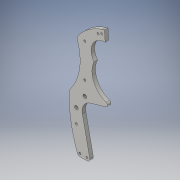
# Autodesk Inventor part: One piece claw 1.0
Saved by Autodesk Inventor 2016 (Build 200138000, 138)
## iProperties
Created: 2016-02-02
Part Number: One piece claw 1.0
Material: Generic
Document SubType Name: Modeling
Designer: Josiah Stark
Density: 1 g/cm^3
Appearance: Default
Author: Josiah Stark
Autodesk Inventor part; units mm, degrees
ref_plane "YZ Plane" through (0, 0, 0) normal (1, 0, 0) x (0, 1, 0)
ref_plane "XZ Plane" through (0, 0, 0) normal (0, 1, 0) x (-1, 0, 0)
ref_plane "XY Plane" through (0, 0, 0) normal (0, 0, 1) x (1, 0, 0)
sketch "Sketch1" plane through (0, 0, 0) normal (0, 0, 1) x (1, 0, 0)
  line L0 (-50.8, -25.4) -> (76.2, -25.4)
  line L1 (76.2, -25.4) -> (76.2, 228.6)
  line L2 (76.2, 228.6) -> (-51.6296, 228.6)
  circle A0 centre (5.08, -4.9022) radius 1.905
  circle A1 centre (-1.27, 63.6778) radius 3.175
  circle A2 centre (13.97, 89.0778) radius 3.175
  arc A3 (23.4649, 83.1687) -> (9.3315, 59.465) centre (29.21, 63.6778) ccw
  arc A4 (0.3002, -6.6225) -> (5.08, -9.9822) centre (5.08, -4.9022) ccw
  line L3 (5.08, -9.9822) -> (17.78, -9.9822)
  arc A5 (17.78, -9.9822) -> (22.7496, -3.849) centre (17.78, -4.9022) ccw
  line L4 (9.3315, 59.465) -> (22.7496, -3.849)
  arc A6 (-14.6784, 83.2471) -> (0.3002, -6.6225) centre (239.2924, 79.3933) ccw
  arc A7 (50.546, 191.9478) -> (30.3529, 151.1401) centre (50.546, 166.5478) ccw
  line L5 (50.546, 191.9478) -> (50.546, 210.9978)
  arc A8 (0.9197, 176.5759) -> (0.1225, 170.7438) centre (6.096, 172.8978) ccw
  arc A9 (50.546, 210.9978) -> (0.9197, 176.5759) centre (73.3878, 125.0824) ccw
  arc A10 (-13.9866, 85.1779) -> (0.1225, 170.7438) centre (-83.5064, 140.5873) ccw
  arc A11 (-13.9866, 85.1779) -> (-14.6784, 83.2471) centre (-11.5038, 83.199) ccw
  circle A12 centre (17.78, -4.9022) radius 1.905
  arc A13 (76.2, 171.1429) -> (75.486, 171.3598) centre (64.77, 134.7978) ccw
  arc A14 (30.3529, 151.1401) -> (52.1919, 98.8339) centre (64.77, 134.7978) ccw
  line L6 (-51.6296, 228.6) -> (-51.6296, 223.5757)
  line L7 (-50.8, -9.9822) -> (-50.8, -25.4)
  line L8 (45.5539, 209.5127) -> (50.546, 210.9978)
  arc A15 (55.9788, 92.7525) -> (55.982, 92.7794) centre (50.3052, 93.4393) ccw
  line L9 (48.0499, 210.2553) -> (50.546, 210.9978)
  line L10 (49.298, 210.6265) -> (50.546, 191.9478)
  line L11 (49.298, 210.6265) -> (49.1762, 210.5903)
  line L12 (49.1762, 210.5903) -> (50.546, 191.9478)
  arc A16 (51.9893, 91.5765) -> (52.1919, 98.8339) centre (50.9341, 95.2375) ccw
  line L13 (45.9382, 89.7529) -> (52.0334, 91.5895)
  line L14 (52.0334, 91.5895) -> (23.4649, 83.1687)
  circle A17 centre (13.97, 114.4778) radius 1.905
  circle A18 centre (13.97, 175.4378) radius 1.905
  circle A19 centre (44.6762, 202.1078) radius 1.905
  circle A20 centre (37.7491, 198.9328) radius 1.905
  circle A21 centre (-1.27, 38.2778) radius 1.905
  point P0 (0, 0)
  point P1 (50.546, 87.6896)
  dimension "d1" = 76.2
  dimension "d2" = 25.4
  dimension "d3" = 228.6
  dimension "d5" = 20.4978
  dimension "d6" = 3.81
  dimension "d7" = 6.35
  dimension "d8" = 89.0778
  dimension "d10" = 6.35
  dimension "d11" = 25.4
  dimension "d12" = 15.24
  dimension "d13" = 30.48
  dimension "d14" = 0
  dimension "d15" = 71.12
  dimension "d16" = 35.56
  dimension "d18" = 40.64
  dimension "d22" = 10.16
  dimension "d23" = 12.7
  dimension "d24" = 10.16
  dimension "d28" = 254
  dimension "d29" = 50.8
  dimension "d30" = 14.224
  dimension "d31" = 31.75
  dimension "d33" = 12.7
  dimension "d34" = 44.45
  dimension "d35" = 38.1
  dimension "d36" = 88.9
  dimension "d37" = 88.9
  dimension "d38" = 3.175
  dimension "d39" = 3.81
  dimension "d43" = 5.08
  dimension "d49" = 11.43
  dimension "d50" = 0.127
  dimension "d53" = 1.27
  dimension "d54" = 19.05
  dimension "d55" = 7.62
  dimension "d56" = 3.81
  dimension "d57" = 25.4
  dimension "d58" = 3.81
  dimension "d59" = 60.96
  dimension "d62" = 3.81
  dimension "d63" = 3.81
  dimension "d64" = 7.62
  dimension "d65" = 10.16
  dimension "d66" = 6.985
  dimension "d67" = 3.81
  dimension "d68" = 25.4
  constraints: 30 end point, 30 point on circle, 22 centre point, 14 tangent, 7 point on line, 3 parallel, 2 coincident, 2 horizontal, 2 midpoint, 1 collinear, 1 line through centre, 1 perpendicular, 1 vertical
  measures "d1" distance from line of point (0, 0) L1
  measures "d2" distance from line of L0 point (0, 0)
  measures "d3" distance from line of point (0, 0) L2
  measures "d5" distance from line of A0.centre L0
  measures "d6" diameter of A0
  measures "d7" diameter of A1
  measures "d8" distance from line of A1.centre L0
  measures "d10" diameter of A2
  measures "d11" vertical distance of A1.centre A2.centre
  measures "d12" horizontal distance of A2.centre A1.centre
  measures "d13" distance of A3.centre A1.centre
  measures "d14" vertical distance of A1.centre A3.centre
  measures "d15" vertical distance of A3.centre A13.centre
  measures "d16" horizontal distance of A13.centre A3.centre
  measures "d18" diameter of A3
  measures "d22" diameter of A4
  measures "d23" distance of L3.start L3.end
  measures "d24" diameter of A5
  measures "d28" radius of A6
  measures "d29" diameter of A7
  measures "d30" horizontal distance of A13.centre A7.centre
  measures "d31" vertical distance of A7.centre A13.centre
  measures "d33" diameter of A8
  measures "d34" distance from line of L5 A8.centre
  measures "d35" vertical distance of L5.end A8.centre
  measures "d36" radius of A9
  measures "d37" radius of A10
  measures "d38" radius of A11
  measures "d39" diameter of A12
  measures "d43" horizontal distance of A4.centre point (0, 0)
  measures "d49" diameter of A15
  measures "d50" distance of L10.start L11.end
  measures "d53" distance from line of L5.end L10
  measures "d54" distance of L5.end L5.start
  measures "d55" diameter of A16
  measures "d56" diameter of A17
  measures "d57" distance of A2.centre A17.centre
  measures "d58" diameter of A18
  measures "d59" distance of A17.centre A18.centre
  measures "d62" diameter of A19
  measures "d63" diameter of A20
  measures "d64" distance of A19.centre A20.centre
  measures "d65" vertical distance of L5.start A19.centre
  measures "d66" vertical distance of L5.start A20.centre
  measures "d67" diameter of A21
  measures "d68" distance of A1.centre A21.centre
extrude "Extrusion6" add sketch "Sketch1" along normal blind 6.35 contours A3 L4 A5 L3 A4 A6 A11 A10 A8 A9 L8 L12 A7 A14 A16 L14 | L12 L8 L10
body "Solid6"
